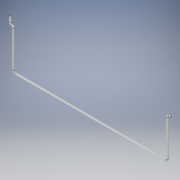
# Autodesk Inventor part: wirePusher
Saved by Autodesk Inventor 2017 (Build 210142000, 142)
## iProperties
Created: 2017-02-21
Part Number: wirePusher
Material: Generic
Document SubType Name: Modeling
Designer: kingb
Density: 1 g/cm^3
Appearance: Default
Author: kingb
Autodesk Inventor part; units mm, degrees
ref_plane "YZ Plane" through (0, 0, 0) normal (1, 0, 0) x (0, 1, 0)
ref_plane "XZ Plane" through (0, 0, 0) normal (0, 1, 0) x (-1, 0, 0)
ref_plane "XY Plane" through (0, 0, 0) normal (0, 0, 1) x (1, 0, 0)
sketch "Sketch1" plane through (0, 0, 0) normal (0, 1, 0) x (-1, 0, 0)
  circle A0 centre (0, 0) radius 1.5875
  dimension "d0" = 3.175
  constraints: 1 centre point, 1 coincident
  measures "d0" diameter of A0
sketch "Sketch2" plane through (0, 0, 0) normal (0, 0, 1) x (1, 0, 0)
  line L0 (0, 0) -> (0, -9.525)
  line L1 (3.175, -12.7) -> (3.175, -12.7)
  line L2 (6.35, -15.875) -> (6.35, -87.3125)
  line L3 (9.525, -90.4875) -> (301.625, -90.4875)
  line L4 (304.8, -87.3125) -> (304.8, -15.875)
  line L5 (307.975, -12.7) -> (311.15, -12.7)
  arc A0 (6.35, -15.875) -> (3.175, -12.7) centre (3.175, -15.875) ccw
  arc A1 (0, -9.525) -> (3.175, -12.7) centre (3.175, -9.525) ccw
  arc A2 (6.35, -87.3125) -> (9.525, -90.4875) centre (9.525, -87.3125) ccw
  arc A3 (301.625, -90.4875) -> (304.8, -87.3125) centre (301.625, -87.3125) ccw
  arc A4 (307.975, -12.7) -> (304.8, -15.875) centre (307.975, -15.875) ccw
  point P0 (0, -12.7)
  point P1 (6.35, -12.7)
  point P2 (6.35, -90.4875)
  point P3 (304.8, -90.4875)
  point P4 (304.8, -12.7)
  dimension "d1" = 12.7
  dimension "d2" = 6.35
  dimension "d3" = 77.7875
  dimension "d4" = 298.45
  dimension "d5" = 6.35
  dimension "d6" = 90
  dimension "d7" = 3.175
  constraints: 12 end point, 10 point on circle, 10 point on line, 10 tangent, 5 centre point, 4 equal radius, 4 perpendicular, 2 vertical
  measures "d1" distance of L0.start point (0, -12.7)
  measures "d2" distance of point (0, -12.7) point (6.35, -12.7)
  measures "d3" distance of point (6.35, -12.7) point (6.35, -90.487)
  measures "d4" distance of point (6.35, -90.487) point (304.8, -90.487)
  measures "d5" distance of point (304.8, -12.7) L5.end
  measures "d6" angle of L4 L5
  measures "d7" radius of A0
sweep "Sweep1" add profiles "Sketch1" path "Sketch2"
body "Solid1"
